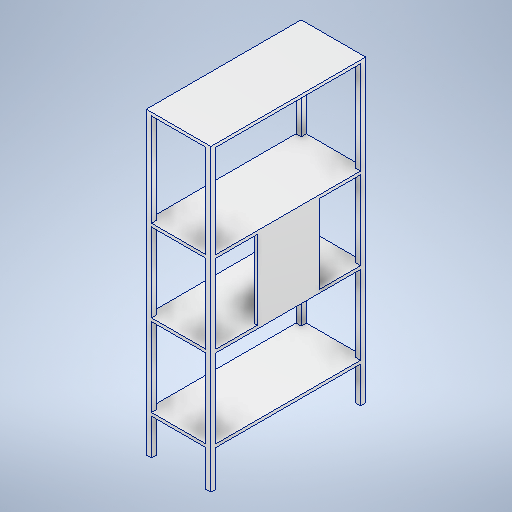
# Autodesk Inventor part: ESTANTERÍA2
Saved by Autodesk Inventor 2025.3 (Build 293356030, 356C)
## iProperties
Created: 2025-12-08
Part Number: ESTANTERÍA2
Material: Aluminio 6061
Document SubType Name: Modeling
Designer: david
Density: 2.7 g/cm^3
Appearance: Aluminio - Plano
Author: david
Autodesk Inventor part; units mm, degrees
ref_plane "YZ Plane" through (0, 0, 0) normal (1, 0, 0) x (0, 1, 0)
ref_plane "XZ Plane" through (0, 0, 0) normal (0, 1, 0) x (-1, 0, 0)
ref_plane "XY Plane" through (0, 0, 0) normal (0, 0, 1) x (1, 0, 0)
sketch "Boceto1" plane through (0, 0, 0) normal (0, 0, 1) x (1, 0, 0)
  line L0 (250, 0) -> (250, 1160)
  line L1 (0, 1160) -> (0, 0)
  line L2 (230, 20) -> (230, 0)
  line L3 (20, 20) -> (20, 0)
  line L4 (230, 0) -> (230, 140)
  line L5 (230, 140) -> (20, 140)
  line L6 (20, 152.5) -> (230, 152.5)
  line L7 (230, 152.5) -> (230, 457.5)
  line L8 (230, 457.5) -> (20, 457.5)
  line L9 (20, 457.5) -> (20, 470)
  line L10 (20, 470) -> (230, 470)
  line L11 (230, 470) -> (230, 457.5)
  line L12 (230, 470) -> (230, 775)
  line L13 (230, 775) -> (20, 775)
  line L14 (20, 775) -> (20, 787.5)
  line L15 (20, 787.5) -> (230, 787.5)
  line L16 (230, 787.5) -> (230, 775)
  line L17 (230, 787.5) -> (230, 1147.5)
  line L18 (230, 1147.5) -> (20, 1147.5)
  line L19 (20, 1160) -> (230, 1160)
  line L20 (230, 1160) -> (230, 1147.5)
  line L21 (0, 0) -> (20, 0)
  line L22 (230, 0) -> (250, 0)
  line L23 (20, 20) -> (20, 140)
  line L24 (230, 140) -> (230, 20)
  line L25 (20, 152.5) -> (20, 457.5)
  line L26 (230, 1147.5) -> (230, 470)
  line L27 (230, 457.5) -> (230, 152.5)
  line L28 (20, 470) -> (20, 775)
  line L29 (20, 787.5) -> (20, 1147.5)
  line L30 (0, 0) -> (529.2462, 0) construction
  line L31 (20, 1160) -> (0, 1160)
  line L32 (230, 1160) -> (250, 1160)
  line L33 (230, 1147.5) -> (250, 1147.5)
  dimension "d5" = 140
  dimension "d6" = 12.5
  dimension "d7" = 305
  dimension "d8" = 12.5
  dimension "d9" = 305
  dimension "d10" = 12.5
  dimension "d11" = 360
  dimension "d13" = 12.5
  dimension "d28" = 1160
  dimension "d29" = 250
  dimension "d30" = 210
  dimension "d31" = 20
  constraints: 68 end point, 19 parallel, 10 perpendicular, 7 horizontal, 3 collinear, 3 point on line
  measures "d5" distance of L2.end L4.end
  measures "d6" distance of L5.end L6.start
  measures "d7" distance of L6.end L7.end
  measures "d8" distance of L8.end L9.end
  measures "d9" distance of L10.end L12.end
  measures "d10" distance of L13.end L14.end
  measures "d11" distance of L17.end L15.end
  measures "d13" distance between parallel lines of L18 L19
  measures "d28" distance from line of L1.end L19
  measures "d29" distance between parallel lines of L0 L1
  measures "d30" distance between parallel lines of L17 L29
  measures "d31" distance between parallel lines of L1 L25
extrude "Extrusión1" add sketch "Boceto1" along normal blind 600 contours L22 L2 L4 L5 L23 L3 L21 L1 L31 L19 L20 L33 L0 | L33 L20 L32 L0 | L16 L13 L14 L15 | L11 L8 L9 L10
sketch "Boceto2" plane through (250, 0, 0) normal (1, 0, 0) x (0, 0, -1)
  line L0 (0, 457.5) -> (0, 152.5) projected
  line L1 (0, 152.5) -> (0, 457.5) projected
  line L2 (0, 0) -> (-600, 0) projected
  line L3 (0, 0) -> (-600, 0) projected
  line L4 (0, 0) -> (-600, 0) projected
  line L5 (0, 0) -> (-600, 0) projected
  line L6 (-600, 140) -> (-600, 0) projected
  line L7 (0, 140) -> (0, 0) projected
  line L8 (0, 0) -> (-600, 0) projected
  line L9 (-600, 140) -> (-600, 0) projected
  line L10 (0, 140) -> (-600, 140) projected
  line L11 (0, 0) -> (-600, 0) projected
  line L12 (0, 0) -> (-600, 0) projected
  line L13 (0, 140) -> (-600, 140) projected
  line L14 (0, 0) -> (0, 140) projected
  line L15 (0, 140) -> (-600, 140) projected
  line L16 (-600, 0) -> (-600, 140) projected
  line L17 (0, 0) -> (-600, 0) projected
  line L18 (0, 140) -> (-600, 140) projected
  line L19 (0, 140) -> (-600, 140) projected
  line L20 (0, 152.5) -> (-600, 152.5) projected
  line L21 (-600, 457.5) -> (-600, 152.5) projected
  line L22 (0, 457.5) -> (0, 152.5) projected
  line L23 (0, 152.5) -> (-600, 152.5) projected
  line L24 (-600, 457.5) -> (-600, 152.5) projected
  line L25 (0, 457.5) -> (-600, 457.5) projected
  line L26 (-600, 152.5) -> (-600, 457.5) projected
  line L27 (0, 152.5) -> (0, 457.5) projected
  line L28 (0, 457.5) -> (-600, 457.5) projected
  line L29 (-600, 152.5) -> (-600, 457.5) projected
  line L30 (0, 152.5) -> (-600, 152.5) projected
  line L31 (0, 0) -> (0, 1160) projected
  line L32 (0, 1160) -> (0, 0) projected
  line L33 (0, 140) -> (0, 0) projected
  line L34 (0, 0) -> (0, 140) projected
  line L35 (0, 1160) -> (0, 0) projected
  line L36 (0, 0) -> (0, 1160) projected
  line L37 (0, 470) -> (0, 775) projected
  line L38 (0, 775) -> (0, 470) projected
  line L39 (0, 152.5) -> (0, 457.5) projected
  line L40 (0, 457.5) -> (0, 152.5) projected
  line L41 (-600, 0) -> (-600, 1160) projected
  line L42 (0, 0) -> (0, 1160) projected
  line L43 (-600, 0) -> (-600, 1160) projected
  line L44 (0, 0) -> (-600, 0) projected
  line L45 (-600, 1160) -> (-600, 0) projected
  line L46 (0, 1160) -> (0, 0) projected
  line L47 (0, 0) -> (-600, 0) projected
  line L48 (-600, 1160) -> (-600, 0) projected
  line L49 (-600, 140) -> (-600, 0) projected
  line L50 (-600, 0) -> (-600, 1160) projected
  line L51 (-600, 1160) -> (-600, 0) projected
  line L52 (-600, 0) -> (-600, 140) projected
  line L53 (-600, 470) -> (-600, 775) projected
  line L54 (-600, 775) -> (-600, 470) projected
  line L55 (-600, 457.5) -> (-600, 152.5) projected
  line L56 (-600, 152.5) -> (-600, 457.5) projected
  line L57 (0, 1600) -> (-600, 1600) projected
  line L58 (0, 152.5) -> (-600, 152.5) projected
  line L59 (0, 152.5) -> (-600, 152.5) projected
  line L60 (0, 152.5) -> (-600, 152.5) projected
  line L61 (0, 0) -> (-600, 0) projected
  line L62 (0, 140) -> (-600, 140) projected
  line L63 (0, 140) -> (0, 0) projected
  line L64 (-600, 0) -> (-600, 140) projected
  line L65 (0, 0) -> (-600, 0) projected
  line L66 (0, 0) -> (0, 140) projected
  line L67 (0, 1160) -> (-600, 1160) projected
  line L68 (0, 1160) -> (-600, 1160) projected
  line L69 (0, 1160) -> (0, 1147.5) projected
  line L70 (0, 1580) -> (-600, 1580) projected
  line L71 (0, 1580) -> (-600, 1580) projected
  line L72 (0, 1580) -> (0, 1160) projected
  line L73 (-600, 1160) -> (-600, 1147.5) projected
  line L74 (-600, 470) -> (-600, 775) projected
  line L75 (0, 457.5) -> (-600, 457.5) projected
  line L76 (0, 457.5) -> (-600, 457.5) projected
  line L77 (0, 457.5) -> (-600, 457.5) projected
  line L78 (0, 457.5) -> (-600, 457.5) projected
  line L79 (0, 470) -> (-600, 470) projected
  line L80 (0, 470) -> (-600, 470) projected
  line L81 (0, 470) -> (-600, 470) projected
  line L82 (-600, 775) -> (-600, 470) projected
  line L83 (0, 775) -> (0, 470) projected
  line L84 (0, 775) -> (0, 470) projected
  line L85 (0, 470) -> (-600, 470) projected
  line L86 (-600, 775) -> (-600, 470) projected
  line L87 (0, 775) -> (-600, 775) projected
  line L88 (0, 470) -> (0, 775) projected
  line L89 (0, 470) -> (0, 775) projected
  line L90 (0, 775) -> (-600, 775) projected
  line L91 (-600, 470) -> (-600, 775) projected
  line L92 (0, 470) -> (-600, 470) projected
  line L93 (0, 470) -> (-600, 470) projected
  line L94 (0, 775) -> (-600, 775) projected
  line L95 (0, 775) -> (-600, 775) projected
  line L96 (0, 775) -> (-600, 775) projected
  line L97 (0, 775) -> (-600, 775) projected
  line L98 (0, 787.5) -> (-600, 787.5) projected
  line L99 (0, 787.5) -> (-600, 787.5) projected
  line L100 (0, 787.5) -> (-600, 787.5) projected
  line L101 (0, 787.5) -> (-600, 787.5) projected
  line L102 (-600, 1147.5) -> (-600, 787.5) projected
  line L103 (-600, 787.5) -> (-600, 1147.5) projected
  line L104 (0, 1147.5) -> (-600, 1147.5) projected
  line L105 (0, 1147.5) -> (0, 787.5) projected
  line L106 (0, 787.5) -> (-600, 787.5) projected
  line L107 (-600, 1147.5) -> (-600, 787.5) projected
  line L108 (0, 1147.5) -> (-600, 1147.5) projected
  line L109 (0, 787.5) -> (0, 1147.5) projected
  line L110 (0, 1147.5) -> (-600, 1147.5) projected
  line L111 (-600, 787.5) -> (-600, 1147.5) projected
  line L112 (0, 787.5) -> (-600, 787.5) projected
  line L113 (0, 1147.5) -> (0, 787.5) projected
  line L114 (0, 787.5) -> (0, 1147.5) projected
  line L115 (0, 1600) -> (-600, 1600) projected
  line L116 (0, 1147.5) -> (-600, 1147.5) projected
  line L117 (0, 1147.5) -> (-600, 1147.5) projected
  line L118 (0, 1147.5) -> (-600, 1147.5) projected
  line L119 (0, 1160) -> (-600, 1160) projected
  line L120 (0, 1160) -> (-600, 1160) projected
  line L121 (0, 787.5) -> (0, 1147.5) projected
  line L122 (-600, 787.5) -> (-600, 1147.5) projected
  line L123 (0, 1580) -> (0, 1160) projected
  line L124 (0, 1160) -> (-600, 1160) projected
  line L125 (-600, 1580) -> (-600, 1160) projected
  line L126 (0, 1580) -> (-600, 1580) projected
  line L127 (0, 1600) -> (-600, 1600) projected
  line L128 (0, 1600) -> (-600, 1600) projected
  line L129 (0, 1580) -> (-600, 1580) projected
  line L130 (0, 1580) -> (-600, 1580) projected
  line L131 (-580, 0) -> (-580, 1600)
  line L132 (-20, 1600) -> (-20, 0)
  line L133 (0, 1160) -> (-600, 1160) projected
  line L134 (0, 1160) -> (-600, 1160) projected
  line L135 (0, 1147.5) -> (-600, 1147.5) projected
  line L136 (0, 787.5) -> (-600, 787.5) projected
  point P0 (-20, 1160)
  point P1 (-20, 1580)
  point P2 (-580, 1580)
  point P3 (-580, 1160)
  point P4 (-20, 787.5)
  point P5 (-20, 1147.5)
  point P6 (-580, 1147.5)
  point P7 (-580, 787.5)
  point P8 (-20, 470)
  point P9 (-20, 775)
  point P10 (-580, 775)
  point P11 (-580, 470)
  point P12 (-20, 152.5)
  point P13 (-20, 457.5)
  point P14 (-580, 457.5)
  point P15 (-580, 152.5)
  point P16 (-20, 140)
  point P17 (-580, 140)
  dimension "d16" = 20
  dimension "d17" = 20
  constraints: 4 end point, 2 vertical, 18 other
  measures "d17" distance of the line from the sketch origin of L132
extrude "Extrusión2" cut sketch "Boceto2" against normal blind 600 contours L132 L20 L131 L25 | L79 L131 L87 L132 | L132 L2 L131 L10 | L98 L131 L104 L132
sketch "Boceto3" plane through (250, 0, 0) normal (1, 0, 0) x (0, 0, -1)
  line L0 (-20, 787.5) -> (-580, 787.5) projected
  line L1 (-20, 1147.5) -> (-580, 1147.5) projected
  line L2 (-420, 787.5) -> (-180, 787.5)
  line L3 (-180, 1147.5) -> (-420, 1147.5)
  line L4 (-580, 787.5) -> (-580, 1147.5) projected
  line L5 (-20, 1147.5) -> (-20, 787.5) projected
  line L6 (-580, 775) -> (-20, 775) projected
  line L7 (-580, 470) -> (-20, 470) projected
  line L8 (-420, 775) -> (-180, 775)
  line L9 (-180, 775) -> (-180, 470)
  line L10 (-180, 470) -> (-420, 470)
  line L11 (-420, 470) -> (-420, 775)
  line L12 (-300, 775) -> (-300, 470)
  line L13 (-20, 775) -> (-20, 470) projected
  point P0 (0, 0)
  dimension "d32" = 240
  dimension "d33" = 160
  constraints: 14 end point, 4 point on line, 3 parallel, 2 horizontal, 2 midpoint, 1 perpendicular
  measures "d32" distance between parallel lines of L9 L11
  measures "d33" distance between parallel lines of L13 L9
extrude "Extrusión3" add sketch "Boceto3" against normal blind 10 contours L6 L12 L7 L11 | L6 L9 L7 L12
